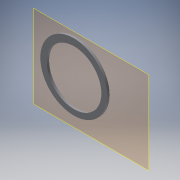
# Autodesk Inventor part: ramp
Saved by Autodesk Inventor 2019 (Build 230136000, 136)
## iProperties
Created: 2019-01-11
Part Number: ramp
Material: Generic
Document SubType Name: Modeling
Designer: jmc
Density: 1 g/cm^3
Appearance: Default
Author: jmc
Autodesk Inventor part; units mm, degrees
ref_plane "YZ Plane" through (0, 0, 0) normal (1, 0, 0) x (0, 1, 0)
ref_plane "XZ Plane" through (0, 0, 0) normal (0, 1, 0) x (-1, 0, 0)
ref_plane "XY Plane" through (0, 0, 0) normal (0, 0, 1) x (1, 0, 0)
ref_plane "Work Plane1" through (0, 0, 0) normal (0, 0, 1) x (1, 0, 0)
sketch "Sketch1" plane through (0, 0, 0) normal (0, 0, 1) x (1, 0, 0)
  circle A0 centre (-11.4142, -28.8682) radius 27.15 construction
  line L0 (-43.1642, -20.886) -> (-43.1642, -36.8503) construction
  arc A1 (-43.1642, -36.8503) -> (-19.3963, -60.6182) centre (-11.4142, -28.8682) ccw construction
  line L1 (-19.3963, -60.6182) -> (-3.4321, -60.6182) construction
  arc A2 (-3.4321, -60.6182) -> (20.3358, -36.8503) centre (-11.4142, -28.8682) ccw construction
  line L2 (20.3358, -36.8503) -> (20.3358, -20.886) construction
  arc A3 (20.3358, -20.886) -> (-3.4321, 2.8818) centre (-11.4142, -28.8682) ccw construction
  line L3 (-3.4321, 2.8818) -> (-19.3963, 2.8818) construction
  arc A4 (-19.3963, 2.8818) -> (-43.1642, -20.886) centre (-11.4142, -28.8682) ccw construction
  circle A5 centre (-11.4142, -28.8682) radius 30
  point P0 (0, 0)
  dimension "d0" = 60
  constraints: 1 centre point, 1 coincident
  measures "d0" diameter of A5
extrude "Extrusion1" add sketch "Sketch1" along normal blind 2
sketch "Sketch2" plane through (-11.4142, -28.8682, 2) normal (0, 0, 1) x (1, 0, 0)
  circle A0 centre (0.2407, -0.5338) radius 24.4145
  circle A1 centre (0, 0) radius 30 projected
  point P0 (11.4142, 28.8682)
  dimension "d3" = 5
  constraints: 1 centre point
extrude "Extrusion2" cut sketch "Sketch2" against normal blind 2 contours A0
body "Solid1"
